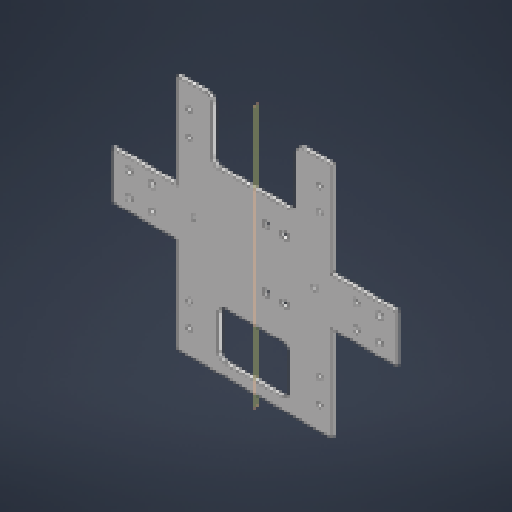
# Autodesk Inventor part: 板子
Saved by Autodesk Inventor 2025 (Build 290162000, 162)
## iProperties
Created: 2026-01-01
Part Number: 板子
Material: 常规
Document SubType Name: Modeling
Designer: XH
Density: 1 g/cm^3
Appearance: 默认
Author: XH
Autodesk Inventor part; units mm, degrees
ref_plane "YZ Plane" through (0, 0, 0) normal (1, 0, 0) x (0, 1, 0)
ref_plane "XZ Plane" through (0, 0, 0) normal (0, 1, 0) x (-1, 0, 0)
ref_plane "XY Plane" through (0, 0, 0) normal (0, 0, 1) x (1, 0, 0)
sketch "草图1" plane through (0, 0, 0) normal (0, 0, 1) x (1, 0, 0)
  line L0 (65, -100) -> (-65, -100)
  line L1 (-65, -100) -> (-65, 100)
  line L2 (-65, 100) -> (65, 100)
  line L3 (65, 100) -> (65, -100)
  line L4 (65, -100) -> (-65, 100) construction
  line L5 (-65, -100) -> (65, 100) construction
  point P0 (0, 0)
  dimension "d0" = 130
  dimension "d1" = 200
  constraints: 12 end point, 2 midpoint, 2 parallel, 1 horizontal, 1 perpendicular
  measures "d0" distance of L1.end L2.end
  measures "d1" distance of L2.end L0.start
extrude "拉伸1" add sketch "草图1" along normal blind 3
sketch "草图2" plane through (0, 0, 3) normal (0, 0, 1) x (1, 0, 0)
  line L0 (120, -20) -> (-120, -20)
  line L1 (-120, -20) -> (-120, 20)
  line L2 (-120, 20) -> (120, 20)
  line L3 (120, 20) -> (120, -20)
  line L4 (120, -20) -> (-120, 20) construction
  line L5 (-120, -20) -> (120, 20) construction
  line L6 (-65, 100) -> (-65, -100) projected
  point P0 (0, 0)
  dimension "d4" = 40
  dimension "d5" = 55
  constraints: 12 end point, 2 midpoint, 2 parallel, 1 horizontal, 1 perpendicular
  measures "d4" distance of L0.end L1.end
  measures "d5" distance between parallel lines of L1 L6
extrude "拉伸2" add sketch "草图2" against normal up to surface (3 mm away)
sketch "草图3" plane through (0, 0, 0) normal (0, 0, -1) x (-1, 0, 0)
  line L0 (120, -20) -> (120, 20) projected
  line L1 (120, 0) -> (-120, 0)
  line L2 (-120, -20) -> (-120, 20) projected
  line L3 (71, 49.9947) -> (71, -50.0053) projected
  line L4 (65, -100) -> (-65, -100) projected
  line L5 (0, -100) -> (0, 7.1575)
  circle A0 centre (86, -10) radius 2.5
  circle A1 centre (106, -10) radius 2.5
  line L6 (65, -20) -> (120, -20) projected
  circle A2 centre (86, 10) radius 2.5
  circle A3 centre (106, 10) radius 2.5
  circle A4 centre (-86, -10) radius 2.5
  circle A5 centre (-106, -10) radius 2.5
  circle A6 centre (-86, 10) radius 2.5
  circle A7 centre (-106, 10) radius 2.5
  point P0 (0, 0)
  dimension "d12" = 5
  dimension "d13" = 5
  dimension "d14" = 20
  dimension "d15" = 10
  dimension "d16" = 15
  constraints: 8 centre point, 6 symmetric about line, 4 end point, 3 midpoint, 1 horizontal alignment, 1 vertical, 6 other
  measures "d12" diameter of A1
  measures "d13" diameter of A0
  measures "d14" distance of A0.centre A1.centre
  measures "d15" distance from line of L6 A0.centre
  measures "d16" distance from line of A0.centre L3
extrude "拉伸3" cut sketch "草图3" against normal blind 10 contours A0 | A1 | A2 | A3 | A4 | A5 | A6 | A7
sketch "草图4" plane through (0, 0, 3) normal (0, 0, 1) x (1, 0, 0)
  line L0 (-30, -90) -> (30, -90)
  line L1 (30, -90) -> (30, -50)
  line L2 (30, -50) -> (-30, -50)
  line L3 (-30, -50) -> (-30, -90)
  line L4 (-30, -90) -> (30, -50) construction
  line L5 (30, -90) -> (-30, -50) construction
  line L6 (-65, -100) -> (65, -100) projected
  point P0 (0, 0)
  point P1 (0, -70)
  dimension "d17" = 10
  dimension "d18" = 60
  dimension "d19" = 40
  constraints: 12 end point, 2 midpoint, 2 parallel, 1 horizontal, 1 perpendicular
  measures "d17" distance between parallel lines of L0 L6
  measures "d18" distance between parallel lines of L3 L1
  measures "d19" distance of L0.end L1.end
extrude "拉伸4" cut sketch "草图4" against normal blind 10
fillet "圆角1" radius 5 4 edges at (30, -90, 1.5) (30, -50, 1.5) (-30, -50, 1.5) (-30, -90, 1.5)
sketch "草图5" plane through (0, 0, 3) normal (0, 0, 1) x (1, 0, 0)
  line L0 (-35, 150) -> (35, 150)
  line L1 (35, 150) -> (35, 50)
  line L2 (35, 50) -> (-35, 50)
  line L3 (-35, 50) -> (-35, 150)
  line L4 (65, 100) -> (-65, 100) projected
  line L5 (-35, 150) -> (35, 50) construction
  line L6 (35, 150) -> (-35, 50) construction
  point P0 (0, 0)
  point P1 (0, 100)
  dimension "d23" = 50
  dimension "d24" = 70
  constraints: 12 end point, 3 midpoint, 2 parallel, 1 horizontal, 1 perpendicular
  measures "d23" distance between parallel lines of L4 L2
  measures "d24" distance of L1.end L2.end
extrude "拉伸5" cut sketch "草图5" against normal blind 10
fillet "圆角2" radius 5 4 edges at (35, 100, 1.5) (35, 50, 1.5) (-35, 50, 1.5) (-35, 100, 1.5)
sketch "草图6" plane through (0, 0, 3) normal (0, 0, 1) x (1, 0, 0)
  line L0 (-120, -20) -> (-120, 20) projected
  line L1 (-120, 3) -> (120, 3)
  line L2 (120, -20) -> (120, 20) projected
  line L3 (-120, 20) -> (-120, -20) projected
  line L4 (-120, -20) -> (-65, -20) projected
  line L5 (-51, -94.6609) -> (-51, 98.803)
  line L6 (-65, -20) -> (-65, -100) projected
  circle A0 centre (-51, 3) radius 2
  point P0 (0, 0)
  dimension "d28" = 23
  dimension "d29" = 14
  dimension "d30" = 4
  constraints: 5 point on line, 4 end point, 1 centre point, 1 perpendicular, 1 vertical
  measures "d28" distance between parallel lines of L1 L4
  measures "d29" distance between parallel lines of L5 L6
  measures "d30" diameter of A0
extrude "拉伸6" cut sketch "草图6" against normal blind 10
ref_plane "工作平面1" through (0, -100, 0) normal (-1, 0, 0) x (0, 0, 1)
mirror "镜像1" about plane through (0, -100, 0) normal (-1, 0, 0) of "拉伸6"
sketch "草图7" plane through (0, 0, 0) normal (0, 0, -1) x (-1, 0, 0)
  line L0 (-8.0092, 31.0916) -> (-13.0092, 31.0916)
  line L1 (-13.0092, 31.0916) -> (-13.0092, 26.0916)
  line L2 (-13.0092, 26.0916) -> (-8.0092, 26.0916)
  line L3 (-8.0092, 26.0916) -> (-8.0092, 31.0916)
  line L4 (-23.0092, 31.0916) -> (-28.0092, 31.0916)
  line L5 (-28.0092, 31.0916) -> (-28.0092, 26.0916)
  line L6 (-28.0092, 26.0916) -> (-23.0092, 26.0916)
  line L7 (-23.0092, 26.0916) -> (-23.0092, 31.0916)
  point P0 (0, 0)
  point P1 (-23.0092, 28.5916)
  point P2 (-13.0092, 28.5916)
  dimension "d33" = 5
  dimension "d34" = 5
  dimension "d35" = 5
  dimension "d36" = 5
  dimension "d37" = 10
  constraints: 16 end point, 4 parallel, 2 horizontal, 2 midpoint, 2 perpendicular, 1 collinear
  measures "d33" distance of L5.end L6.end
  measures "d34" distance of L1.end L2.end
  measures "d35" distance of L2.end L0.start
  measures "d36" distance of L6.end L4.start
  measures "d37" distance of point (-23.009, 28.592) point (-13.009, 28.592)
extrude "拉伸7" cut sketch "草图7" against normal blind 10
pattern_linear "矩形阵列1" count 2 spacing 50 along (0, -1, 0) of "拉伸7"
sketch "草图8" plane through (0, 0, 0) normal (0, 0, -1) x (-1, 0, 0)
  circle A0 centre (-55, -60) radius 2
  line L0 (65, -100) -> (-65, -100) projected
  line L1 (-65, -100) -> (-65, -20) projected
  circle A1 centre (-55, -80) radius 2
  line L2 (-55, -100) -> (-55, -60)
  line L3 (0, 0) -> (-45.6081, 0)
  line L4 (0, 0) -> (0, -68.1904)
  circle A2 centre (55, -60) radius 2
  line L5 (65, -100) -> (65, -20)
  circle A3 centre (55, -80) radius 2
  circle A4 centre (-55, 60) radius 2
  circle A5 centre (-55, 80) radius 2
  circle A6 centre (55, 60) radius 2
  circle A7 centre (55, 80) radius 2
  point P0 (-65, 100)
  point P1 (-55, 100)
  point P2 (0, 68.1904)
  dimension "d43" = 40
  dimension "d45" = 4
  dimension "d46" = 10
  dimension "d47" = 4
  dimension "d48" = 20
  constraints: 10 symmetric about line, 8 centre point, 8 end point, 2 vertical, 1 horizontal, 1 midpoint, 1 point on line, 6 other
  measures "d43" distance from line of L0 L2.end
  measures "d45" diameter of A0
  measures "d46" distance from line of L1 L2.end
  measures "d47" diameter of A1
  measures "d48" distance of L2.end A1.centre
extrude "拉伸8" cut sketch "草图8" against normal blind 10
